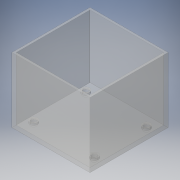
# Autodesk Inventor part: Attachable top
Saved by Autodesk Inventor 2016 (Build 200138000, 138)
## iProperties
Created: 2015-09-15
Part Number: Attachable top
Material: PET Plastic
Document SubType Name: Modeling
Designer: rossmosier
Density: 1.541 g/cm^3
Appearance: Polycarbonate - Clear
Author: rossmosier
Autodesk Inventor part; units mm, degrees
ref_plane "YZ Plane" through (0, 0, 0) normal (1, 0, 0) x (0, 1, 0)
ref_plane "XZ Plane" through (0, 0, 0) normal (0, 1, 0) x (-1, 0, 0)
ref_plane "XY Plane" through (0, 0, 0) normal (0, 0, 1) x (1, 0, 0)
sketch "Sketch1" plane through (0, 0, 0) normal (0, 1, 0) x (-1, 0, 0)
  line L0 (0, 0) -> (-457.2, 0)
  line L1 (-457.2, 0) -> (-457.2, -457.2)
  line L2 (-457.2, -457.2) -> (0, -457.2)
  line L3 (0, -457.2) -> (0, 0)
  dimension "d0" = 457.2
  dimension "d1" = 457.2
  constraints: 8 end point, 2 parallel, 1 horizontal, 1 perpendicular
  measures "d0" distance of L2.end L1.end
  measures "d1" distance of L1.end L0.end
extrude "Extrusion1" add sketch "Sketch1" along normal blind 381
sketch "Sketch2" plane through (0, 381, 0) normal (0, 1, 0) x (1, 0, 0)
  line L0 (0, 0) -> (457.2, 0) projected
  line L1 (457.2, 0) -> (457.2, 457.2) projected
  line L2 (457.2, 457.2) -> (0, 457.2) projected
  line L3 (0, 457.2) -> (0, 0) projected
  line L4 (12.7, 12.7) -> (444.5, 12.7)
  line L5 (444.5, 12.7) -> (444.5, 444.5)
  line L6 (444.5, 444.5) -> (12.7, 444.5)
  line L7 (12.7, 444.5) -> (12.7, 12.7)
  dimension "d4" = 12.7
  constraints: 8 end point, 3 other
  measures "d4" distance between parallel lines of L3 L7
extrude "Extrusion2" cut sketch "Sketch2" against normal blind 368.3 contours L7 L6 L5 L4
sketch "Sketch3" plane through (0, 0, 0) normal (0, -1, 0) x (1, 0, 0)
  line L0 (0, 0) -> (457.2, 0) projected
  line L1 (0, -457.2) -> (0, 0) projected
  line L2 (457.2, -457.2) -> (0, -457.2) projected
  line L3 (457.2, 0) -> (457.2, -457.2) projected
  line L4 (457.2, 0) -> (406.4, 0) construction
  line L5 (0, 0) -> (457.2, 0) construction
  line L6 (406.4, 0) -> (406.4, -76.2) construction
  circle A0 centre (406.4, -76.2) radius 15.875
  line L7 (457.2, 0) -> (457.2, -457.2) construction
  line L8 (457.2, -228.6) -> (0, -228.6) construction
  line L9 (228.6, 0) -> (228.6, -457.2) construction
  circle A1 centre (406.4, -381) radius 15.875
  circle A2 centre (50.8, -381) radius 15.875
  circle A3 centre (50.8, -76.2) radius 15.875
  point P0 (228.6, -228.6)
  dimension "d7" = 50.8
  dimension "d8" = 76.2
  dimension "d9" = 31.75
  constraints: 8 end point, 5 midpoint, 4 centre point, 3 symmetric about line, 1 coincident, 1 perpendicular, 1 point on line, 3 other
  measures "d7" distance of L0.end L4.end
  measures "d8" distance of L4.end L6.end
  measures "d9" diameter of A0
extrude "Extrusion3" cut sketch "Sketch3" against normal blind 25.4 contours A0 | A1 | A2 | A3
sketch "Sketch5" plane through (0, 12.7, 0) normal (0, 1, 0) x (1, 0, 0)
  circle A0 centre (50.8, 381) radius 15.875 projected
  circle A1 centre (406.4, 76.2) radius 15.875 projected
  circle A2 centre (406.4, 381) radius 15.875 projected
  circle A3 centre (50.8, 76.2) radius 15.875 projected
  line L0 (444.5, 12.7) -> (12.7, 12.7) projected
  line L1 (444.5, 444.5) -> (444.5, 12.7) projected
  line L2 (12.7, 444.5) -> (444.5, 444.5) projected
  line L3 (12.7, 12.7) -> (12.7, 444.5) projected
  circle A4 centre (50.8, 381) radius 22.225
  circle A5 centre (406.4, 381) radius 22.225
  circle A6 centre (50.8, 76.2) radius 22.225
  circle A7 centre (406.4, 76.2) radius 22.225
  point P0 (0, 0)
  dimension "d19" = 6.35
  dimension "d20" = 6.35
  dimension "d21" = 6.35
  dimension "d22" = 6.35
  constraints: 4 centre point
  measures "d19" radial gap between concentric circles of A0 A4
  measures "d20" radial gap between concentric circles of A2 A5
  measures "d21" radial gap between concentric circles of A3 A6
  measures "d22" radial gap between concentric circles of A1 A7
extrude "Extrusion5" add sketch "Sketch5" along normal blind 12.7 contours A4 | A5 | A6 | A7
body "Solid1"
